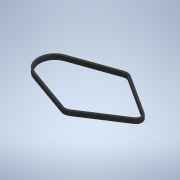
# Autodesk Inventor part: GT2_TimingBelt Base
Saved by Autodesk Inventor 2020.4 (Build 244396010, 396A)
## iProperties
Created: 2021-10-18
Part Number: GT2_TimingBelt Base
Material: Rubber
Document SubType Name: Modeling
Designer: justi
Density: 0.93 g/cm^3
Appearance: Rubber - Black
Author: justi
Autodesk Inventor part; units mm, degrees
ref_plane "YZ Plane" through (0, 0, 0) normal (1, 0, 0) x (0, 1, 0)
ref_plane "XZ Plane" through (0, 0, 0) normal (0, 1, 0) x (-1, 0, 0)
ref_plane "XY Plane" through (0, 0, 0) normal (0, 0, 1) x (1, 0, 0)
sketch "Sketch1" plane through (0, 0, 0) normal (0, 1, 0) x (-1, 0, 0)
  arc A0 (-3.262608, 5.035414) -> (-3.262608, -5.035414) centre (0, 0) ccw
  line L0 (0, 0) -> (47.5, 0) construction
  line L1 (47.5, 0) -> (47.5, -27.5) construction
  line L2 (47.5, 0) -> (47.5, 27.5) construction
  arc A1 (42.74203, -34.843311) -> (50.42338, -35.747202) centre (47.5, -27.5) ccw
  arc A2 (50.42338, 35.747202) -> (42.74203, 34.843311) centre (47.5, 27.5) ccw
  line L3 (47.5, 0) -> (95, 0) construction
  arc A3 (101.281091, -17.719703) -> (101.281091, 17.719703) centre (95, 0) ccw
  line L4 (101.281091, 17.719703) -> (50.42338, 35.747202)
  line L5 (101.281091, -17.719703) -> (50.42338, -35.747202)
  line L6 (42.74203, -34.843311) -> (-3.262608, -5.035414)
  line L7 (42.74203, 34.843311) -> (-3.262608, 5.035414)
  dimension "d0" = 12
  dimension "d1" = 47.5
  dimension "d2" = 27.5
  dimension "d3" = 27.5
  dimension "d4" = 17.5
  dimension "d5" = 17.5
  dimension "d6" = 47.5
  dimension "d7" = 37.6
  constraints: 16 end point, 8 point on circle, 8 tangent, 4 centre point, 4 coincident, 2 horizontal, 2 vertical
  measures "d0" diameter of A0
  measures "d1" distance of L0.start L0.end
  measures "d2" distance of L0.end L1.end
  measures "d3" distance of L0.end L2.end
  measures "d4" diameter of A1
  measures "d5" diameter of A2
  measures "d6" distance of L0.end L3.end
  measures "d7" diameter of A3
sketch "Sketch2" plane through (0, 0, 0) normal (0, 0, 1) x (1, 0, 0)
  line L0 (0, 0) -> (6, 0)
  line L1 (5, 2.5) -> (5, -2.5)
  line L2 (5, -2.5) -> (7, -2.5)
  line L3 (7, -2.5) -> (7, 2.5)
  line L4 (7, 2.5) -> (5, 2.5)
  line L5 (5, 2.5) -> (7, -2.5) construction
  line L6 (5, -2.5) -> (7, 2.5) construction
  dimension "d8" = 6
  dimension "d9" = 2
  dimension "d10" = 5
  constraints: 14 end point, 2 midpoint, 2 parallel, 1 horizontal, 1 perpendicular, 1 vertical
  measures "d8" distance of L0.start L0.end
  measures "d9" distance of L2.end L1.end
  measures "d10" distance of L2.end L3.end
sweep "Sweep1" add profiles "Sketch2" path "Sketch1" path curves A0 L6 A1 L5 A3 L4 A2 L7
body "Solid1"
